Autodesk Fusion 360 part; units mm, degrees
(part 3 of 7)
sketch "スケッチ8" plane through (0, 0, 15) normal (0, 0, 1) x (-1, 0, 0)
  line L0 (-22, 92.5) -> (-17.5, 92.5)
  line L1 (-17.5, 92.5) -> (-15, 95)
  line L2 (-15, 95) -> (-10, 95)
  line L3 (-10, 95) -> (-7.5, 92.5)
  line L4 (-7.5, 92.5) -> (-3, 92.5)
  arc A0 (-3, 91.5) -> (-3, 92.5) centre (-3, 92) ccw
  line L5 (-3, 91.5) -> (-7.5, 91.5)
  line L6 (-7.5, 91.5) -> (-10, 94)
  line L7 (-10, 94) -> (-15, 94)
  line L8 (-15, 94) -> (-17.5, 91.5)
  line L9 (-17.5, 91.5) -> (-22, 91.5)
  arc A1 (-22, 92.5) -> (-22, 91.5) centre (-22, 92) ccw
  arc A2 (-9.9466, 90.4891) -> (-15.0533, 90.4891) centre (-12.5, 89.9985) ccw
  line L10 (-9.9466, 90.4891) -> (-3, 90.4891)
  arc A3 (-3, 89.508) -> (-3, 90.4891) centre (-2.9907, 89.9985) ccw
  line L11 (-3, 89.508) -> (-9.9467, 89.508)
  arc A4 (-15.0532, 89.508) -> (-9.9467, 89.508) centre (-12.5, 89.9985) ccw
  line L12 (-15.0532, 89.508) -> (-22, 89.508)
  arc A5 (-22, 90.4891) -> (-22, 89.508) centre (-22.0093, 89.9985) ccw
  line L13 (-22, 90.4891) -> (-15.0533, 90.4891)
  line L14 (-257, 90.4891) -> (-250.0533, 90.4891)
  arc A6 (-244.9466, 90.4891) -> (-250.0533, 90.4891) centre (-247.5, 89.9985) ccw
  line L15 (-244.9466, 90.4891) -> (-238, 90.4891)
  arc A7 (-238, 89.508) -> (-238, 90.4891) centre (-237.9907, 89.9985) ccw
  line L16 (-238, 89.508) -> (-244.9467, 89.508)
  arc A8 (-250.0532, 89.508) -> (-244.9467, 89.508) centre (-247.5, 89.9985) ccw
  line L17 (-250.0532, 89.508) -> (-257, 89.508)
  arc A9 (-257, 90.4891) -> (-257, 89.508) centre (-257.0093, 89.9985) ccw
  line L18 (-257, 92.5) -> (-252.5, 92.5)
  line L19 (-252.5, 92.5) -> (-250, 95)
  line L20 (-250, 95) -> (-245, 95)
  line L21 (-245, 95) -> (-242.5, 92.5)
  line L22 (-242.5, 92.5) -> (-238, 92.5)
  arc A10 (-238, 91.5) -> (-238, 92.5) centre (-238, 92) ccw
  line L23 (-238, 91.5) -> (-242.5, 91.5)
  line L24 (-242.5, 91.5) -> (-245, 94)
  line L25 (-245, 94) -> (-250, 94)
  line L26 (-250, 94) -> (-252.5, 91.5)
  line L27 (-252.5, 91.5) -> (-257, 91.5)
  arc A11 (-257, 92.5) -> (-257, 91.5) centre (-257, 92) ccw
  line L28 (-5.5, 97) -> (-254.5, 97)
  arc A12 (-254.5, 97) -> (-260.1618, 89.0141) centre (-254.5, 91) ccw
  arc A13 (-257.5, 70) -> (-260.1618, 89.0141) centre (-326.7422, 70) ccw
  spline S0 degree 3 poles (-257.5, 70) (-257.4682, 70) (-257.4042, 70.0035) (-257.3084, 70.0191) (-257.2129, 70.045) (-257.0835, 70.094) (-256.9569, 70.1632) (-256.8341, 70.249) (-256.7405, 70.3242) (-256.6475, 70.4088) (-256.555, 70.5025) (-256.4632, 70.6049) (-256.3391, 70.7561) (-256.1865, 70.9661) (-256.0102, 71.2437) (-255.8375, 71.5492) (-255.6685, 71.8799) (-255.5036, 72.2332) (-255.3429, 72.6062) (-255.1866, 72.9962) (-255.0347, 73.4004) (-254.8872, 73.8162) (-254.6952, 74.3858) (-254.4671, 75.111) (-254.2087, 75.9886) (-253.9612, 76.8646) (-253.7209, 77.7274) (-253.4836, 78.5677) (-253.2448, 79.3779) (-253, 80.1518) (-252.745, 80.8848) (-252.4757, 81.5734) (-252.189, 82.2149) (-251.8824, 82.8074) (-251.5542, 83.3498) (-251.2032, 83.8412) (-250.8288, 84.2811) (-250.4306, 84.6692) (-250.1457, 84.8961) (-250, 85) knots -1.723892 -1.723892 -1.723892 -1.723892 -1.714347 -1.704698 -1.694847 -1.684702 -1.663244 -1.65179 -1.639799 -1.627239 -1.614089 -1.600335 -1.585971 -1.555429 -1.522524 -1.487384 -1.450184 -1.411129 -1.370442 -1.328355 -1.285102 -1.240909 -1.195991 -1.104775 -1.012886 -0.921529 -0.831696 -0.744179 -0.659582 -0.578332 -0.500694 -0.426786 -0.356594 -0.289994 -0.226758 -0.166571 -0.109035 -0.053684 0 0 0 0
  spline S1 degree 5 poles (-250, 85) (-249.8618, 84.9014) (-249.5912, 84.691) (-249.2034, 84.3357) (-248.7221, 83.7824) (-248.1794, 82.9585) (-247.6925, 82.0039) (-247.2547, 80.9239) (-246.8537, 79.7274) (-246.4726, 78.4298) (-246.0928, 77.0547) (-245.6957, 75.6366) (-245.2655, 74.223) (-244.7912, 72.8764) (-244.2698, 71.6789) (-243.7063, 70.7262) (-243.1114, 70.1082) (-242.5, 69.8927) (-241.8886, 70.1082) (-241.2937, 70.7262) (-240.7302, 71.6789) (-240.2088, 72.8764) (-239.7345, 74.223) (-239.3043, 75.6366) (-238.9072, 77.0547) (-238.5274, 78.4298) (-238.1463, 79.7274) (-237.7453, 80.9239) (-237.3075, 82.0039) (-236.8206, 82.9585) (-236.2779, 83.7824) (-235.7966, 84.3357) (-235.4088, 84.691) (-235.1382, 84.9014) (-235, 85) knots -1 -1 -1 -1 -1 -1 -0.966667 -0.933333 -0.9 -0.866667 -0.833333 -0.8 -0.766667 -0.733333 -0.7 -0.666667 -0.633333 -0.6 -0.566667 -0.533333 -0.5 -0.466667 -0.433333 -0.4 -0.366667 -0.333333 -0.3 -0.266667 -0.233333 -0.2 -0.166667 -0.133333 -0.1 -0.066667 -0.033333 0 0 0 0 0 0
  spline S2 degree 5 poles (-235, 85) (-234.8618, 84.9014) (-234.5912, 84.691) (-234.2034, 84.3357) (-233.7221, 83.7824) (-233.1794, 82.9585) (-232.6925, 82.0039) (-232.2547, 80.9239) (-231.8537, 79.7274) (-231.4726, 78.4298) (-231.0928, 77.0547) (-230.6957, 75.6366) (-230.2655, 74.223) (-229.7912, 72.8764) (-229.2698, 71.6789) (-228.7063, 70.7262) (-228.1114, 70.1082) (-227.5, 69.8927) (-226.8886, 70.1082) (-226.2937, 70.7262) (-225.7302, 71.6789) (-225.2088, 72.8764) (-224.7345, 74.223) (-224.3043, 75.6366) (-223.9072, 77.0547) (-223.5274, 78.4298) (-223.1463, 79.7274) (-222.7453, 80.9239) (-222.3075, 82.0039) (-221.8206, 82.9585) (-221.2779, 83.7824) (-220.7966, 84.3357) (-220.4088, 84.691) (-220.1382, 84.9014) (-220, 85) knots -1 -1 -1 -1 -1 -1 -0.966667 -0.933333 -0.9 -0.866667 -0.833333 -0.8 -0.766667 -0.733333 -0.7 -0.666667 -0.633333 -0.6 -0.566667 -0.533333 -0.5 -0.466667 -0.433333 -0.4 -0.366667 -0.333333 -0.3 -0.266667 -0.233333 -0.2 -0.166667 -0.133333 -0.1 -0.066667 -0.033333 0 0 0 0 0 0
  spline S3 degree 5 poles (-220, 85) (-219.8618, 84.9014) (-219.5912, 84.691) (-219.2034, 84.3357) (-218.7221, 83.7824) (-218.1794, 82.9585) (-217.6925, 82.0039) (-217.2547, 80.9239) (-216.8537, 79.7274) (-216.4726, 78.4298) (-216.0928, 77.0547) (-215.6957, 75.6366) (-215.2655, 74.223) (-214.7912, 72.8764) (-214.2698, 71.6789) (-213.7063, 70.7262) (-213.1114, 70.1082) (-212.5, 69.8927) (-211.8886, 70.1082) (-211.2937, 70.7262) (-210.7302, 71.6789) (-210.2088, 72.8764) (-209.7345, 74.223) (-209.3043, 75.6366) (-208.9072, 77.0547) (-208.5274, 78.4298) (-208.1463, 79.7274) (-207.7453, 80.9239) (-207.3075, 82.0039) (-206.8206, 82.9585) (-206.2779, 83.7824) (-205.7966, 84.3357) (-205.4088, 84.691) (-205.1382, 84.9014) (-205, 85) knots -1 -1 -1 -1 -1 -1 -0.966667 -0.933333 -0.9 -0.866667 -0.833333 -0.8 -0.766667 -0.733333 -0.7 -0.666667 -0.633333 -0.6 -0.566667 -0.533333 -0.5 -0.466667 -0.433333 -0.4 -0.366667 -0.333333 -0.3 -0.266667 -0.233333 -0.2 -0.166667 -0.133333 -0.1 -0.066667 -0.033333 0 0 0 0 0 0
  spline S4 degree 5 poles (-205, 85) (-204.8618, 84.9014) (-204.5912, 84.691) (-204.2034, 84.3357) (-203.7221, 83.7824) (-203.1794, 82.9585) (-202.6925, 82.0039) (-202.2547, 80.9239) (-201.8537, 79.7274) (-201.4726, 78.4298) (-201.0928, 77.0547) (-200.6957, 75.6366) (-200.2655, 74.223) (-199.7912, 72.8764) (-199.2698, 71.6789) (-198.7063, 70.7262) (-198.1114, 70.1082) (-197.5, 69.8927) (-196.8886, 70.1082) (-196.2937, 70.7262) (-195.7302, 71.6789) (-195.2088, 72.8764) (-194.7345, 74.223) (-194.3043, 75.6366) (-193.9072, 77.0547) (-193.5274, 78.4298) (-193.1463, 79.7274) (-192.7453, 80.9239) (-192.3075, 82.0039) (-191.8206, 82.9585) (-191.2779, 83.7824) (-190.7966, 84.3357) (-190.4088, 84.691) (-190.1382, 84.9014) (-190, 85) knots -1 -1 -1 -1 -1 -1 -0.966667 -0.933333 -0.9 -0.866667 -0.833333 -0.8 -0.766667 -0.733333 -0.7 -0.666667 -0.633333 -0.6 -0.566667 -0.533333 -0.5 -0.466667 -0.433333 -0.4 -0.366667 -0.333333 -0.3 -0.266667 -0.233333 -0.2 -0.166667 -0.133333 -0.1 -0.066667 -0.033333 0 0 0 0 0 0
  spline S5 degree 5 poles (-190, 85) (-189.8618, 84.9014) (-189.5912, 84.691) (-189.2034, 84.3357) (-188.7221, 83.7824) (-188.1794, 82.9585) (-187.6925, 82.0039) (-187.2547, 80.9239) (-186.8537, 79.7274) (-186.4726, 78.4298) (-186.0928, 77.0547) (-185.6957, 75.6366) (-185.2655, 74.223) (-184.7912, 72.8764) (-184.2698, 71.6789) (-183.7063, 70.7262) (-183.1114, 70.1082) (-182.5, 69.8927) (-181.8886, 70.1082) (-181.2937, 70.7262) (-180.7302, 71.6789) (-180.2088, 72.8764) (-179.7345, 74.223) (-179.3043, 75.6366) (-178.9072, 77.0547) (-178.5274, 78.4298) (-178.1463, 79.7274) (-177.7453, 80.9239) (-177.3075, 82.0039) (-176.8206, 82.9585) (-176.2779, 83.7824) (-175.7966, 84.3357) (-175.4088, 84.691) (-175.1382, 84.9014) (-175, 85) knots -1 -1 -1 -1 -1 -1 -0.966667 -0.933333 -0.9 -0.866667 -0.833333 -0.8 -0.766667 -0.733333 -0.7 -0.666667 -0.633333 -0.6 -0.566667 -0.533333 -0.5 -0.466667 -0.433333 -0.4 -0.366667 -0.333333 -0.3 -0.266667 -0.233333 -0.2 -0.166667 -0.133333 -0.1 -0.066667 -0.033333 0 0 0 0 0 0
  spline S6 degree 5 poles (-175, 85) (-174.8618, 84.9014) (-174.5912, 84.691) (-174.2034, 84.3357) (-173.7221, 83.7824) (-173.1794, 82.9585) (-172.6925, 82.0039) (-172.2547, 80.9239) (-171.8537, 79.7274) (-171.4726, 78.4298) (-171.0928, 77.0547) (-170.6957, 75.6366) (-170.2655, 74.223) (-169.7912, 72.8764) (-169.2698, 71.6789) (-168.7063, 70.7262) (-168.1114, 70.1082) (-167.5, 69.8927) (-166.8886, 70.1082) (-166.2937, 70.7262) (-165.7302, 71.6789) (-165.2088, 72.8764) (-164.7345, 74.223) (-164.3043, 75.6366) (-163.9072, 77.0547) (-163.5274, 78.4298) (-163.1463, 79.7274) (-162.7453, 80.9239) (-162.3075, 82.0039) (-161.8206, 82.9585) (-161.2779, 83.7824) (-160.7966, 84.3357) (-160.4088, 84.691) (-160.1382, 84.9014) (-160, 85) knots -1 -1 -1 -1 -1 -1 -0.966667 -0.933333 -0.9 -0.866667 -0.833333 -0.8 -0.766667 -0.733333 -0.7 -0.666667 -0.633333 -0.6 -0.566667 -0.533333 -0.5 -0.466667 -0.433333 -0.4 -0.366667 -0.333333 -0.3 -0.266667 -0.233333 -0.2 -0.166667 -0.133333 -0.1 -0.066667 -0.033333 0 0 0 0 0 0
  spline S7 degree 5 poles (-160, 85) (-159.8618, 84.9014) (-159.5912, 84.691) (-159.2034, 84.3357) (-158.7221, 83.7824) (-158.1794, 82.9585) (-157.6925, 82.0039) (-157.2547, 80.9239) (-156.8537, 79.7274) (-156.4726, 78.4298) (-156.0928, 77.0547) (-155.6957, 75.6366) (-155.2655, 74.223) (-154.7912, 72.8764) (-154.2698, 71.6789) (-153.7063, 70.7262) (-153.1114, 70.1082) (-152.5, 69.8927) (-151.8886, 70.1082) (-151.2937, 70.7262) (-150.7302, 71.6789) (-150.2088, 72.8764) (-149.7345, 74.223) (-149.3043, 75.6366) (-148.9072, 77.0547) (-148.5274, 78.4298) (-148.1463, 79.7274) (-147.7453, 80.9239) (-147.3075, 82.0039) (-146.8206, 82.9585) (-146.2779, 83.7824) (-145.7966, 84.3357) (-145.4088, 84.691) (-145.1382, 84.9014) (-145, 85) knots -1 -1 -1 -1 -1 -1 -0.966667 -0.933333 -0.9 -0.866667 -0.833333 -0.8 -0.766667 -0.733333 -0.7 -0.666667 -0.633333 -0.6 -0.566667 -0.533333 -0.5 -0.466667 -0.433333 -0.4 -0.366667 -0.333333 -0.3 -0.266667 -0.233333 -0.2 -0.166667 -0.133333 -0.1 -0.066667 -0.033333 0 0 0 0 0 0
  spline S8 degree 5 poles (-145, 85) (-144.8618, 84.9014) (-144.5912, 84.691) (-144.2034, 84.3357) (-143.7221, 83.7824) (-143.1794, 82.9585) (-142.6925, 82.0039) (-142.2547, 80.9239) (-141.8537, 79.7274) (-141.4726, 78.4298) (-141.0928, 77.0547) (-140.6957, 75.6366) (-140.2655, 74.223) (-139.7912, 72.8764) (-139.2698, 71.6789) (-138.7063, 70.7262) (-138.1114, 70.1082) (-137.5, 69.8927) (-136.8886, 70.1082) (-136.2937, 70.7262) (-135.7302, 71.6789) (-135.2088, 72.8764) (-134.7345, 74.223) (-134.3043, 75.6366) (-133.9072, 77.0547) (-133.5274, 78.4298) (-133.1463, 79.7274) (-132.7453, 80.9239) (-132.3075, 82.0039) (-131.8206, 82.9585) (-131.2779, 83.7824) (-130.7966, 84.3357) (-130.4088, 84.691) (-130.1382, 84.9014) (-130, 85) knots -1 -1 -1 -1 -1 -1 -0.966667 -0.933333 -0.9 -0.866667 -0.833333 -0.8 -0.766667 -0.733333 -0.7 -0.666667 -0.633333 -0.6 -0.566667 -0.533333 -0.5 -0.466667 -0.433333 -0.4 -0.366667 -0.333333 -0.3 -0.266667 -0.233333 -0.2 -0.166667 -0.133333 -0.1 -0.066667 -0.033333 0 0 0 0 0 0
  spline S9 degree 5 poles (-130, 85) (-129.8618, 84.9014) (-129.5912, 84.691) (-129.2034, 84.3357) (-128.7221, 83.7824) (-128.1794, 82.9585) (-127.6925, 82.0039) (-127.2547, 80.9239) (-126.8537, 79.7274) (-126.4726, 78.4298) (-126.0928, 77.0547) (-125.6957, 75.6366) (-125.2655, 74.223) (-124.7912, 72.8764) (-124.2698, 71.6789) (-123.7063, 70.7262) (-123.1114, 70.1082) (-122.5, 69.8927) (-121.8886, 70.1082) (-121.2937, 70.7262) (-120.7302, 71.6789) (-120.2088, 72.8764) (-119.7345, 74.223) (-119.3043, 75.6366) (-118.9072, 77.0547) (-118.5274, 78.4298) (-118.1463, 79.7274) (-117.7453, 80.9239) (-117.3075, 82.0039) (-116.8206, 82.9585) (-116.2779, 83.7824) (-115.7966, 84.3357) (-115.4088, 84.691) (-115.1382, 84.9014) (-115, 85) knots -1 -1 -1 -1 -1 -1 -0.966667 -0.933333 -0.9 -0.866667 -0.833333 -0.8 -0.766667 -0.733333 -0.7 -0.666667 -0.633333 -0.6 -0.566667 -0.533333 -0.5 -0.466667 -0.433333 -0.4 -0.366667 -0.333333 -0.3 -0.266667 -0.233333 -0.2 -0.166667 -0.133333 -0.1 -0.066667 -0.033333 0 0 0 0 0 0
  spline S10 degree 5 poles (-115, 85) (-114.8618, 84.9014) (-114.5912, 84.691) (-114.2034, 84.3357) (-113.7221, 83.7824) (-113.1794, 82.9585) (-112.6925, 82.0039) (-112.2547, 80.9239) (-111.8537, 79.7274) (-111.4726, 78.4298) (-111.0928, 77.0547) (-110.6957, 75.6366) (-110.2655, 74.223) (-109.7912, 72.8764) (-109.2698, 71.6789) (-108.7063, 70.7262) (-108.1114, 70.1082) (-107.5, 69.8927) (-106.8886, 70.1082) (-106.2937, 70.7262) (-105.7302, 71.6789) (-105.2088, 72.8764) (-104.7345, 74.223) (-104.3043, 75.6366) (-103.9072, 77.0547) (-103.5274, 78.4298) (-103.1463, 79.7274) (-102.7453, 80.9239) (-102.3075, 82.0039) (-101.8206, 82.9585) (-101.2779, 83.7824) (-100.7966, 84.3357) (-100.4088, 84.691) (-100.1382, 84.9014) (-100, 85) knots -1 -1 -1 -1 -1 -1 -0.966667 -0.933333 -0.9 -0.866667 -0.833333 -0.8 -0.766667 -0.733333 -0.7 -0.666667 -0.633333 -0.6 -0.566667 -0.533333 -0.5 -0.466667 -0.433333 -0.4 -0.366667 -0.333333 -0.3 -0.266667 -0.233333 -0.2 -0.166667 -0.133333 -0.1 -0.066667 -0.033333 0 0 0 0 0 0
  spline S11 degree 5 poles (-100, 85) (-99.8618, 84.9014) (-99.5912, 84.691) (-99.2034, 84.3357) (-98.7221, 83.7824) (-98.1794, 82.9585) (-97.6925, 82.0039) (-97.2547, 80.9239) (-96.8537, 79.7274) (-96.4726, 78.4298) (-96.0928, 77.0547) (-95.6957, 75.6366) (-95.2655, 74.223) (-94.7912, 72.8764) (-94.2698, 71.6789) (-93.7063, 70.7262) (-93.1114, 70.1082) (-92.5, 69.8927) (-91.8886, 70.1082) (-91.2937, 70.7262) (-90.7302, 71.6789) (-90.2088, 72.8764) (-89.7345, 74.223) (-89.3043, 75.6366) (-88.9072, 77.0547) (-88.5274, 78.4298) (-88.1463, 79.7274) (-87.7453, 80.9239) (-87.3075, 82.0039) (-86.8206, 82.9585) (-86.2779, 83.7824) (-85.7966, 84.3357) (-85.4088, 84.691) (-85.1382, 84.9014) (-85, 85) knots -1 -1 -1 -1 -1 -1 -0.966667 -0.933333 -0.9 -0.866667 -0.833333 -0.8 -0.766667 -0.733333 -0.7 -0.666667 -0.633333 -0.6 -0.566667 -0.533333 -0.5 -0.466667 -0.433333 -0.4 -0.366667 -0.333333 -0.3 -0.266667 -0.233333 -0.2 -0.166667 -0.133333 -0.1 -0.066667 -0.033333 0 0 0 0 0 0
  spline S12 degree 5 poles (-85, 85) (-84.8618, 84.9014) (-84.5912, 84.691) (-84.2034, 84.3357) (-83.7221, 83.7824) (-83.1794, 82.9585) (-82.6925, 82.0039) (-82.2547, 80.9239) (-81.8537, 79.7274) (-81.4726, 78.4298) (-81.0928, 77.0547) (-80.6957, 75.6366) (-80.2655, 74.223) (-79.7912, 72.8764) (-79.2698, 71.6789) (-78.7063, 70.7262) (-78.1114, 70.1082) (-77.5, 69.8927) (-76.8886, 70.1082) (-76.2937, 70.7262) (-75.7302, 71.6789) (-75.2088, 72.8764) (-74.7345, 74.223) (-74.3043, 75.6366) (-73.9072, 77.0547) (-73.5274, 78.4298) (-73.1463, 79.7274) (-72.7453, 80.9239) (-72.3075, 82.0039) (-71.8206, 82.9585) (-71.2779, 83.7824) (-70.7966, 84.3357) (-70.4088, 84.691) (-70.1382, 84.9014) (-70, 85) knots -1 -1 -1 -1 -1 -1 -0.966667 -0.933333 -0.9 -0.866667 -0.833333 -0.8 -0.766667 -0.733333 -0.7 -0.666667 -0.633333 -0.6 -0.566667 -0.533333 -0.5 -0.466667 -0.433333 -0.4 -0.366667 -0.333333 -0.3 -0.266667 -0.233333 -0.2 -0.166667 -0.133333 -0.1 -0.066667 -0.033333 0 0 0 0 0 0
  spline S13 degree 5 poles (-70, 85) (-69.8618, 84.9014) (-69.5912, 84.691) (-69.2034, 84.3357) (-68.7221, 83.7824) (-68.1794, 82.9585) (-67.6925, 82.0039) (-67.2547, 80.9239) (-66.8537, 79.7274) (-66.4726, 78.4298) (-66.0928, 77.0547) (-65.6957, 75.6366) (-65.2655, 74.223) (-64.7912, 72.8764) (-64.2698, 71.6789) (-63.7063, 70.7262) (-63.1114, 70.1082) (-62.5, 69.8927) (-61.8886, 70.1082) (-61.2937, 70.7262) (-60.7302, 71.6789) (-60.2088, 72.8764) (-59.7345, 74.223) (-59.3043, 75.6366) (-58.9072, 77.0547) (-58.5274, 78.4298) (-58.1463, 79.7274) (-57.7453, 80.9239) (-57.3075, 82.0039) (-56.8206, 82.9585) (-56.2779, 83.7824) (-55.7966, 84.3357) (-55.4088, 84.691) (-55.1382, 84.9014) (-55, 85) knots -1 -1 -1 -1 -1 -1 -0.966667 -0.933333 -0.9 -0.866667 -0.833333 -0.8 -0.766667 -0.733333 -0.7 -0.666667 -0.633333 -0.6 -0.566667 -0.533333 -0.5 -0.466667 -0.433333 -0.4 -0.366667 -0.333333 -0.3 -0.266667 -0.233333 -0.2 -0.166667 -0.133333 -0.1 -0.066667 -0.033333 0 0 0 0 0 0
  spline S14 degree 5 poles (-55, 85) (-54.8618, 84.9014) (-54.5912, 84.691) (-54.2034, 84.3357) (-53.7221, 83.7824) (-53.1794, 82.9585) (-52.6925, 82.0039) (-52.2547, 80.9239) (-51.8537, 79.7274) (-51.4726, 78.4298) (-51.0928, 77.0547) (-50.6957, 75.6366) (-50.2655, 74.223) (-49.7912, 72.8764) (-49.2698, 71.6789) (-48.7063, 70.7262) (-48.1114, 70.1082) (-47.5, 69.8927) (-46.8886, 70.1082) (-46.2937, 70.7262) (-45.7302, 71.6789) (-45.2088, 72.8764) (-44.7345, 74.223) (-44.3043, 75.6366) (-43.9072, 77.0547) (-43.5274, 78.4298) (-43.1463, 79.7274) (-42.7453, 80.9239) (-42.3075, 82.0039) (-41.8206, 82.9585) (-41.2779, 83.7824) (-40.7966, 84.3357) (-40.4088, 84.691) (-40.1382, 84.9014) (-40, 85) knots -1 -1 -1 -1 -1 -1 -0.966667 -0.933333 -0.9 -0.866667 -0.833333 -0.8 -0.766667 -0.733333 -0.7 -0.666667 -0.633333 -0.6 -0.566667 -0.533333 -0.5 -0.466667 -0.433333 -0.4 -0.366667 -0.333333 -0.3 -0.266667 -0.233333 -0.2 -0.166667 -0.133333 -0.1 -0.066667 -0.033333 0 0 0 0 0 0
  spline S15 degree 5 poles (-40, 85) (-39.8618, 84.9014) (-39.5912, 84.691) (-39.2034, 84.3357) (-38.7221, 83.7824) (-38.1794, 82.9585) (-37.6925, 82.0039) (-37.2547, 80.9239) (-36.8537, 79.7274) (-36.4726, 78.4298) (-36.0928, 77.0547) (-35.6957, 75.6366) (-35.2655, 74.223) (-34.7912, 72.8764) (-34.2698, 71.6789) (-33.7063, 70.7262) (-33.1114, 70.1082) (-32.5, 69.8927) (-31.8886, 70.1082) (-31.2937, 70.7262) (-30.7302, 71.6789) (-30.2088, 72.8764) (-29.7345, 74.223) (-29.3043, 75.6366) (-28.9072, 77.0547) (-28.5274, 78.4298) (-28.1463, 79.7274) (-27.7453, 80.9239) (-27.3075, 82.0039) (-26.8206, 82.9585) (-26.2779, 83.7824) (-25.7966, 84.3357) (-25.4088, 84.691) (-25.1382, 84.9014) (-25, 85) knots -1 -1 -1 -1 -1 -1 -0.966667 -0.933333 -0.9 -0.866667 -0.833333 -0.8 -0.766667 -0.733333 -0.7 -0.666667 -0.633333 -0.6 -0.566667 -0.533333 -0.5 -0.466667 -0.433333 -0.4 -0.366667 -0.333333 -0.3 -0.266667 -0.233333 -0.2 -0.166667 -0.133333 -0.1 -0.066667 -0.033333 0 0 0 0 0 0
  spline S16 degree 5 poles (-25, 85) (-24.8618, 84.9014) (-24.5912, 84.691) (-24.2034, 84.3357) (-23.7221, 83.7824) (-23.1794, 82.9585) (-22.6925, 82.0039) (-22.2547, 80.9239) (-21.8537, 79.7274) (-21.4726, 78.4298) (-21.0928, 77.0547) (-20.6957, 75.6366) (-20.2655, 74.223) (-19.7912, 72.8764) (-19.2698, 71.6789) (-18.7063, 70.7262) (-18.1114, 70.1082) (-17.5, 69.8927) (-16.8886, 70.1082) (-16.2937, 70.7262) (-15.7302, 71.6789) (-15.2088, 72.8764) (-14.7345, 74.223) (-14.3043, 75.6366) (-13.9072, 77.0547) (-13.5274, 78.4298) (-13.1463, 79.7274) (-12.7453, 80.9239) (-12.3075, 82.0039) (-11.8206, 82.9585) (-11.2779, 83.7824) (-10.7966, 84.3357) (-10.4088, 84.691) (-10.1382, 84.9014) (-10, 85) knots -1 -1 -1 -1 -1 -1 -0.966667 -0.933333 -0.9 -0.866667 -0.833333 -0.8 -0.766667 -0.733333 -0.7 -0.666667 -0.633333 -0.6 -0.566667 -0.533333 -0.5 -0.466667 -0.433333 -0.4 -0.366667 -0.333333 -0.3 -0.266667 -0.233333 -0.2 -0.166667 -0.133333 -0.1 -0.066667 -0.033333 0 0 0 0 0 0
  spline S17 degree 5 poles (-10, 85) (-9.8618, 84.9014) (-9.5912, 84.691) (-9.2034, 84.3357) (-8.7221, 83.7824) (-8.1794, 82.9585) (-7.6925, 82.0039) (-7.2547, 80.9239) (-6.8537, 79.7274) (-6.4726, 78.4298) (-6.0928, 77.0547) (-5.6957, 75.6366) (-5.2655, 74.223) (-4.7912, 72.8764) (-4.2698, 71.6789) (-3.7063, 70.7262) (-3.2304, 70.2318) (-2.866, 70.0421) (-2.622, 70) (-2.5, 70) knots -1 -1 -1 -1 -1 -1 -0.966667 -0.933333 -0.9 -0.866667 -0.833333 -0.8 -0.766667 -0.733333 -0.7 -0.666667 -0.633333 -0.6 -0.566667 -0.533333 -0.5 -0.5 -0.5 -0.5 -0.5 -0.5
  arc A14 (-0.0354, 88.5224) -> (-2.5, 70) centre (93.3503, 66.6714) ccw
  arc A15 (-0.0354, 88.5224) -> (-5.5, 97) centre (-5.5, 91) ccw
  spline S18 degree 3 poles (-40, 87.4565) (-39.6129, 87.1804) (-39.2258, 86.9044) (-38.8387, 86.6283) (-37.4048, 85.6057) (-36.3881, 84.0523) (-35.6468, 82.2521) (-34.9554, 80.5733) (-34.4675, 78.6373) (-33.9195, 76.7225) (-33.5808, 75.5389) (-33.2149, 74.3638) (-32.8326, 73.4325) (-32.7208, 73.1603) (-32.6088, 72.9111) (-32.5, 72.6931) knots -1.056001 -1.056001 -1.056001 -1.056001 -1 -1 -1 -0.851292 -0.851292 -0.851292 -0.71262 -0.71262 -0.71262 -0.626906 -0.626906 -0.626906 -0.601856 -0.601856 -0.601856 -0.601856
  spline S19 degree 3 poles (-32.5, 72.6931) (-32.0881, 73.5183) (-31.6514, 74.7828) (-31.2668, 76.0817) (-30.7129, 77.9522) (-30.237, 79.9069) (-29.6002, 81.6203) (-28.9085, 83.4814) (-27.986, 85.1149) (-26.6355, 86.2591) (-26.4823, 86.3889) (-26.3242, 86.5122) (-26.1613, 86.6283) (-25.7742, 86.9044) (-25.3871, 87.1804) (-25, 87.4565) knots -0.398144 -0.398144 -0.398144 -0.398144 -0.30293 -0.30293 -0.30293 -0.165823 -0.165823 -0.165823 -0.016893 -0.016893 -0.016893 0 0 0 0.056001 0.056001 0.056001 0.056001
  spline S20 degree 3 poles (-25, 87.4565) (-24.6129, 87.1804) (-24.2258, 86.9044) (-23.8387, 86.6283) (-22.4048, 85.6057) (-21.3881, 84.0523) (-20.6468, 82.2521) (-19.9554, 80.5733) (-19.4675, 78.6373) (-18.9195, 76.7225) (-18.5808, 75.5389) (-18.2149, 74.3638) (-17.8326, 73.4325) (-17.7208, 73.1603) (-17.6088, 72.9111) (-17.5, 72.6931) knots -1.056001 -1.056001 -1.056001 -1.056001 -1 -1 -1 -0.851292 -0.851292 -0.851292 -0.71262 -0.71262 -0.71262 -0.626906 -0.626906 -0.626906 -0.601856 -0.601856 -0.601856 -0.601856
  arc A16 (-2.3166, 87.5) -> (-4.0079, 77.0332) centre (93.3503, 66.6714) ccw
  arc A17 (-255.8863, 77.4088) -> (-257.6718, 87.4565) centre (-326.7422, 70) ccw
  spline S21 degree 3 poles (-242.5, 72.6931) (-242.0881, 73.5183) (-241.6514, 74.7828) (-241.2668, 76.0817) (-240.7129, 77.9522) (-240.237, 79.9069) (-239.6002, 81.6203) (-238.9085, 83.4814) (-237.986, 85.1149) (-236.6355, 86.2591) (-236.4823, 86.3889) (-236.3242, 86.5122) (-236.1613, 86.6283) (-235.7742, 86.9044) (-235.3871, 87.1804) (-235, 87.4565) knots -0.398144 -0.398144 -0.398144 -0.398144 -0.30293 -0.30293 -0.30293 -0.165823 -0.165823 -0.165823 -0.016893 -0.016893 -0.016893 0 0 0 0.056001 0.056001 0.056001 0.056001
  spline S22 degree 3 poles (-235, 87.4565) (-234.6129, 87.1804) (-234.2258, 86.9044) (-233.8387, 86.6283) (-232.4048, 85.6057) (-231.3881, 84.0523) (-230.6468, 82.2521) (-229.9554, 80.5733) (-229.4675, 78.6373) (-228.9195, 76.7225) (-228.5808, 75.5389) (-228.2149, 74.3638) (-227.8326, 73.4325) (-227.7208, 73.1603) (-227.6088, 72.9111) (-227.5, 72.6931) knots -1.056001 -1.056001 -1.056001 -1.056001 -1 -1 -1 -0.851292 -0.851292 -0.851292 -0.71262 -0.71262 -0.71262 -0.626906 -0.626906 -0.626906 -0.601856 -0.601856 -0.601856 -0.601856
  spline S23 degree 3 poles (-227.5, 72.6931) (-227.0881, 73.5183) (-226.6514, 74.7828) (-226.2668, 76.0817) (-225.7129, 77.9522) (-225.237, 79.9069) (-224.6002, 81.6203) (-223.9085, 83.4814) (-222.986, 85.1149) (-221.6355, 86.2591) (-221.4823, 86.3889) (-221.3242, 86.5122) (-221.1613, 86.6283) (-220.7742, 86.9044) (-220.3871, 87.1804) (-220, 87.4565) knots -0.398144 -0.398144 -0.398144 -0.398144 -0.30293 -0.30293 -0.30293 -0.165823 -0.165823 -0.165823 -0.016893 -0.016893 -0.016893 0 0 0 0.056001 0.056001 0.056001 0.056001
  spline S24 degree 3 poles (-220, 87.4565) (-219.6129, 87.1804) (-219.2258, 86.9044) (-218.8387, 86.6283) (-217.4048, 85.6057) (-216.3881, 84.0523) (-215.6468, 82.2521) (-214.9554, 80.5733) (-214.4675, 78.6373) (-213.9195, 76.7225) (-213.5808, 75.5389) (-213.2149, 74.3638) (-212.8326, 73.4325) (-212.7208, 73.1603) (-212.6088, 72.9111) (-212.5, 72.6931) knots -1.056001 -1.056001 -1.056001 -1.056001 -1 -1 -1 -0.851292 -0.851292 -0.851292 -0.71262 -0.71262 -0.71262 -0.626906 -0.626906 -0.626906 -0.601856 -0.601856 -0.601856 -0.601856
  spline S25 degree 3 poles (-212.5, 72.6931) (-212.0881, 73.5183) (-211.6514, 74.7828) (-211.2668, 76.0817) (-210.7129, 77.9522) (-210.237, 79.9069) (-209.6002, 81.6203) (-208.9085, 83.4814) (-207.986, 85.1149) (-206.6355, 86.2591) (-206.4823, 86.3889) (-206.3242, 86.5122) (-206.1613, 86.6283) (-205.7742, 86.9044) (-205.3871, 87.1804) (-205, 87.4565) knots -0.398144 -0.398144 -0.398144 -0.398144 -0.30293 -0.30293 -0.30293 -0.165823 -0.165823 -0.165823 -0.016893 -0.016893 -0.016893 0 0 0 0.056001 0.056001 0.056001 0.056001
  spline S26 degree 3 poles (-205, 87.4565) (-204.6129, 87.1804) (-204.2258, 86.9044) (-203.8387, 86.6283) (-202.4048, 85.6057) (-201.3881, 84.0523) (-200.6468, 82.2521) (-199.9554, 80.5733) (-199.4675, 78.6373) (-198.9195, 76.7225) (-198.5808, 75.5389) (-198.2149, 74.3638) (-197.8326, 73.4325) (-197.7208, 73.1603) (-197.6088, 72.9111) (-197.5, 72.6931) knots -1.056001 -1.056001 -1.056001 -1.056001 -1 -1 -1 -0.851292 -0.851292 -0.851292 -0.71262 -0.71262 -0.71262 -0.626906 -0.626906 -0.626906 -0.601856 -0.601856 -0.601856 -0.601856
  spline S27 degree 3 poles (-197.5, 72.6931) (-197.0881, 73.5183) (-196.6514, 74.7828) (-196.2668, 76.0817) (-195.7129, 77.9522) (-195.237, 79.9069) (-194.6002, 81.6203) (-193.9085, 83.4814) (-192.986, 85.1149) (-191.6355, 86.2591) (-191.4823, 86.3889) (-191.3242, 86.5122) (-191.1613, 86.6283) (-190.7742, 86.9044) (-190.3871, 87.1804) (-190, 87.4565) knots -0.398144 -0.398144 -0.398144 -0.398144 -0.30293 -0.30293 -0.30293 -0.165823 -0.165823 -0.165823 -0.016893 -0.016893 -0.016893 0 0 0 0.056001 0.056001 0.056001 0.056001
  spline S28 degree 3 poles (-190, 87.4565) (-189.6129, 87.1804) (-189.2258, 86.9044) (-188.8387, 86.6283) (-187.4048, 85.6057) (-186.3881, 84.0523) (-185.6468, 82.2521) (-184.9554, 80.5733) (-184.4675, 78.6373) (-183.9195, 76.7225) (-183.5808, 75.5389) (-183.2149, 74.3638) (-182.8326, 73.4325) (-182.7208, 73.1603) (-182.6088, 72.9111) (-182.5, 72.6931) knots -1.056001 -1.056001 -1.056001 -1.056001 -1 -1 -1 -0.851292 -0.851292 -0.851292 -0.71262 -0.71262 -0.71262 -0.626906 -0.626906 -0.626906 -0.601856 -0.601856 -0.601856 -0.601856
  spline S29 degree 3 poles (-182.5, 72.6931) (-182.0881, 73.5183) (-181.6514, 74.7828) (-181.2668, 76.0817) (-180.7129, 77.9522) (-180.237, 79.9069) (-179.6002, 81.6203) (-178.9085, 83.4814) (-177.986, 85.1149) (-176.6355, 86.2591) (-176.4823, 86.3889) (-176.3242, 86.5122) (-176.1613, 86.6283) (-175.7742, 86.9044) (-175.3871, 87.1804) (-175, 87.4565) knots -0.398144 -0.398144 -0.398144 -0.398144 -0.30293 -0.30293 -0.30293 -0.165823 -0.165823 -0.165823 -0.016893 -0.016893 -0.016893 0 0 0 0.056001 0.056001 0.056001 0.056001
  spline S30 degree 3 poles (-175, 87.4565) (-174.6129, 87.1804) (-174.2258, 86.9044) (-173.8387, 86.6283) (-172.4048, 85.6057) (-171.3881, 84.0523) (-170.6468, 82.2521) (-169.9554, 80.5733) (-169.4675, 78.6373) (-168.9195, 76.7225) (-168.5808, 75.5389) (-168.2149, 74.3638) (-167.8326, 73.4325) (-167.7208, 73.1603) (-167.6088, 72.9111) (-167.5, 72.6931) knots -1.056001 -1.056001 -1.056001 -1.056001 -1 -1 -1 -0.851292 -0.851292 -0.851292 -0.71262 -0.71262 -0.71262 -0.626906 -0.626906 -0.626906 -0.601856 -0.601856 -0.601856 -0.601856
  spline S31 degree 3 poles (-167.5, 72.6931) (-167.0881, 73.5183) (-166.6514, 74.7828) (-166.2668, 76.0817) (-165.7129, 77.9522) (-165.237, 79.9069) (-164.6002, 81.6203) (-163.9085, 83.4814) (-162.986, 85.1149) (-161.6355, 86.2591) (-161.4823, 86.3889) (-161.3242, 86.5122) (-161.1613, 86.6283) (-160.7742, 86.9044) (-160.3871, 87.1804) (-160, 87.4565) knots -0.398144 -0.398144 -0.398144 -0.398144 -0.30293 -0.30293 -0.30293 -0.165823 -0.165823 -0.165823 -0.016893 -0.016893 -0.016893 0 0 0 0.056001 0.056001 0.056001 0.056001
  spline S32 degree 3 poles (-160, 87.4565) (-159.6129, 87.1804) (-159.2258, 86.9044) (-158.8387, 86.6283) (-157.4048, 85.6057) (-156.3881, 84.0523) (-155.6468, 82.2521) (-154.9554, 80.5733) (-154.4675, 78.6373) (-153.9195, 76.7225) (-153.5808, 75.5389) (-153.2149, 74.3638) (-152.8326, 73.4325) (-152.7208, 73.1603) (-152.6088, 72.9111) (-152.5, 72.6931) knots -1.056001 -1.056001 -1.056001 -1.056001 -1 -1 -1 -0.851292 -0.851292 -0.851292 -0.71262 -0.71262 -0.71262 -0.626906 -0.626906 -0.626906 -0.601856 -0.601856 -0.601856 -0.601856
  spline S33 degree 3 poles (-152.5, 72.6931) (-152.0881, 73.5183) (-151.6514, 74.7828) (-151.2668, 76.0817) (-150.7129, 77.9522) (-150.237, 79.9069) (-149.6002, 81.6203) (-148.9085, 83.4814) (-147.986, 85.1149) (-146.6355, 86.2591) (-146.4823, 86.3889) (-146.3242, 86.5122) (-146.1613, 86.6283) (-145.7742, 86.9044) (-145.3871, 87.1804) (-145, 87.4565) knots -0.398144 -0.398144 -0.398144 -0.398144 -0.30293 -0.30293 -0.30293 -0.165823 -0.165823 -0.165823 -0.016893 -0.016893 -0.016893 0 0 0 0.056001 0.056001 0.056001 0.056001
  spline S34 degree 3 poles (-145, 87.4565) (-144.6129, 87.1804) (-144.2258, 86.9044) (-143.8387, 86.6283) (-142.4048, 85.6057) (-141.3881, 84.0523) (-140.6468, 82.2521) (-139.9554, 80.5733) (-139.4675, 78.6373) (-138.9195, 76.7225) (-138.5808, 75.5389) (-138.2149, 74.3638) (-137.8326, 73.4325) (-137.7208, 73.1603) (-137.6088, 72.9111) (-137.5, 72.6931) knots -1.056001 -1.056001 -1.056001 -1.056001 -1 -1 -1 -0.851292 -0.851292 -0.851292 -0.71262 -0.71262 -0.71262 -0.626906 -0.626906 -0.626906 -0.601856 -0.601856 -0.601856 -0.601856
  spline S35 degree 3 poles (-137.5, 72.6931) (-137.0881, 73.5183) (-136.6514, 74.7828) (-136.2668, 76.0817) (-135.7129, 77.9522) (-135.237, 79.9069) (-134.6002, 81.6203) (-133.9085, 83.4814) (-132.986, 85.1149) (-131.6355, 86.2591) (-131.4823, 86.3889) (-131.3242, 86.5122) (-131.1613, 86.6283) (-130.7742, 86.9044) (-130.3871, 87.1804) (-130, 87.4565) knots -0.398144 -0.398144 -0.398144 -0.398144 -0.30293 -0.30293 -0.30293 -0.165823 -0.165823 -0.165823 -0.016893 -0.016893 -0.016893 0 0 0 0.056001 0.056001 0.056001 0.056001
  spline S36 degree 3 poles (-130, 87.4565) (-129.6129, 87.1804) (-129.2258, 86.9044) (-128.8387, 86.6283) (-127.4048, 85.6057) (-126.3881, 84.0523) (-125.6468, 82.2521) (-124.9554, 80.5733) (-124.4675, 78.6373) (-123.9195, 76.7225) (-123.5808, 75.5389) (-123.2149, 74.3638) (-122.8326, 73.4325) (-122.7208, 73.1603) (-122.6088, 72.9111) (-122.5, 72.6931) knots -1.056001 -1.056001 -1.056001 -1.056001 -1 -1 -1 -0.851292 -0.851292 -0.851292 -0.71262 -0.71262 -0.71262 -0.626906 -0.626906 -0.626906 -0.601856 -0.601856 -0.601856 -0.601856
  spline S37 degree 3 poles (-122.5, 72.6931) (-122.0881, 73.5183) (-121.6514, 74.7828) (-121.2668, 76.0817) (-120.7129, 77.9522) (-120.237, 79.9069) (-119.6002, 81.6203) (-118.9085, 83.4814) (-117.986, 85.1149) (-116.6355, 86.2591) (-116.4823, 86.3889) (-116.3242, 86.5122) (-116.1613, 86.6283) (-115.7742, 86.9044) (-115.3871, 87.1804) (-115, 87.4565) knots -0.398144 -0.398144 -0.398144 -0.398144 -0.30293 -0.30293 -0.30293 -0.165823 -0.165823 -0.165823 -0.016893 -0.016893 -0.016893 0 0 0 0.056001 0.056001 0.056001 0.056001
  spline S38 degree 3 poles (-115, 87.4565) (-114.6129, 87.1804) (-114.2258, 86.9044) (-113.8387, 86.6283) (-112.4048, 85.6057) (-111.3881, 84.0523) (-110.6468, 82.2521) (-109.9554, 80.5733) (-109.4675, 78.6373) (-108.9195, 76.7225) (-108.5808, 75.5389) (-108.2149, 74.3638) (-107.8326, 73.4325) (-107.7208, 73.1603) (-107.6088, 72.9111) (-107.5, 72.6931) knots -1.056001 -1.056001 -1.056001 -1.056001 -1 -1 -1 -0.851292 -0.851292 -0.851292 -0.71262 -0.71262 -0.71262 -0.626906 -0.626906 -0.626906 -0.601856 -0.601856 -0.601856 -0.601856
  spline S39 degree 3 poles (-107.5, 72.6931) (-107.0881, 73.5183) (-106.6514, 74.7828) (-106.2668, 76.0817) (-105.7129, 77.9522) (-105.237, 79.9069) (-104.6002, 81.6203) (-103.9085, 83.4814) (-102.986, 85.1149) (-101.6355, 86.2591) (-101.4823, 86.3889) (-101.3242, 86.5122) (-101.1613, 86.6283) (-100.7742, 86.9044) (-100.3871, 87.1804) (-100, 87.4565) knots -0.398144 -0.398144 -0.398144 -0.398144 -0.30293 -0.30293 -0.30293 -0.165823 -0.165823 -0.165823 -0.016893 -0.016893 -0.016893 0 0 0 0.056001 0.056001 0.056001 0.056001
  spline S40 degree 3 poles (-100, 87.4565) (-99.6129, 87.1804) (-99.2258, 86.9044) (-98.8387, 86.6283) (-97.4048, 85.6057) (-96.3881, 84.0523) (-95.6468, 82.2521) (-94.9554, 80.5733) (-94.4675, 78.6373) (-93.9195, 76.7225) (-93.5808, 75.5389) (-93.2149, 74.3638) (-92.8326, 73.4325) (-92.7208, 73.1603) (-92.6088, 72.9111) (-92.5, 72.6931) knots -1.056001 -1.056001 -1.056001 -1.056001 -1 -1 -1 -0.851292 -0.851292 -0.851292 -0.71262 -0.71262 -0.71262 -0.626906 -0.626906 -0.626906 -0.601856 -0.601856 -0.601856 -0.601856
  spline S41 degree 3 poles (-92.5, 72.6931) (-92.0881, 73.5183) (-91.6514, 74.7828) (-91.2668, 76.0817) (-90.7129, 77.9522) (-90.237, 79.9069) (-89.6002, 81.6203) (-88.9085, 83.4814) (-87.986, 85.1149) (-86.6355, 86.2591) (-86.4823, 86.3889) (-86.3242, 86.5122) (-86.1613, 86.6283) (-85.7742, 86.9044) (-85.3871, 87.1804) (-85, 87.4565) knots -0.398144 -0.398144 -0.398144 -0.398144 -0.30293 -0.30293 -0.30293 -0.165823 -0.165823 -0.165823 -0.016893 -0.016893 -0.016893 0 0 0 0.056001 0.056001 0.056001 0.056001
  spline S42 degree 3 poles (-85, 87.4565) (-84.6129, 87.1804) (-84.2258, 86.9044) (-83.8387, 86.6283) (-82.4048, 85.6057) (-81.3881, 84.0523) (-80.6468, 82.2521) (-79.9554, 80.5733) (-79.4675, 78.6373) (-78.9195, 76.7225) (-78.5808, 75.5389) (-78.2149, 74.3638) (-77.8326, 73.4325) (-77.7208, 73.1603) (-77.6088, 72.9111) (-77.5, 72.6931) knots -1.056001 -1.056001 -1.056001 -1.056001 -1 -1 -1 -0.851292 -0.851292 -0.851292 -0.71262 -0.71262 -0.71262 -0.626906 -0.626906 -0.626906 -0.601856 -0.601856 -0.601856 -0.601856
  spline S43 degree 3 poles (-77.5, 72.6931) (-77.0881, 73.5183) (-76.6514, 74.7828) (-76.2668, 76.0817) (-75.7129, 77.9522) (-75.237, 79.9069) (-74.6002, 81.6203) (-73.9085, 83.4814) (-72.986, 85.1149) (-71.6355, 86.2591) (-71.4823, 86.3889) (-71.3242, 86.5122) (-71.1613, 86.6283) (-70.7742, 86.9044) (-70.3871, 87.1804) (-70, 87.4565) knots -0.398144 -0.398144 -0.398144 -0.398144 -0.30293 -0.30293 -0.30293 -0.165823 -0.165823 -0.165823 -0.016893 -0.016893 -0.016893 0 0 0 0.056001 0.056001 0.056001 0.056001
  spline S44 degree 3 poles (-70, 87.4565) (-69.6129, 87.1804) (-69.2258, 86.9044) (-68.8387, 86.6283) (-67.4048, 85.6057) (-66.3881, 84.0523) (-65.6468, 82.2521) (-64.9554, 80.5733) (-64.4675, 78.6373) (-63.9195, 76.7225) (-63.5808, 75.5389) (-63.2149, 74.3638) (-62.8326, 73.4325) (-62.7208, 73.1603) (-62.6088, 72.9111) (-62.5, 72.6931) knots -1.056001 -1.056001 -1.056001 -1.056001 -1 -1 -1 -0.851292 -0.851292 -0.851292 -0.71262 -0.71262 -0.71262 -0.626906 -0.626906 -0.626906 -0.601856 -0.601856 -0.601856 -0.601856
  spline S45 degree 3 poles (-62.5, 72.6931) (-62.0881, 73.5183) (-61.6514, 74.7828) (-61.2668, 76.0817) (-60.7129, 77.9522) (-60.237, 79.9069) (-59.6002, 81.6203) (-58.9085, 83.4814) (-57.986, 85.1149) (-56.6355, 86.2591) (-56.4823, 86.3889) (-56.3242, 86.5122) (-56.1613, 86.6283) (-55.7742, 86.9044) (-55.3871, 87.1804) (-55, 87.4565) knots -0.398144 -0.398144 -0.398144 -0.398144 -0.30293 -0.30293 -0.30293 -0.165823 -0.165823 -0.165823 -0.016893 -0.016893 -0.016893 0 0 0 0.056001 0.056001 0.056001 0.056001
  spline S46 degree 3 poles (-55, 87.4565) (-54.6129, 87.1804) (-54.2258, 86.9044) (-53.8387, 86.6283) (-52.4048, 85.6057) (-51.3881, 84.0523) (-50.6468, 82.2521) (-49.9554, 80.5733) (-49.4675, 78.6373) (-48.9195, 76.7225) (-48.5808, 75.5389) (-48.2149, 74.3638) (-47.8326, 73.4325) (-47.7208, 73.1603) (-47.6088, 72.9111) (-47.5, 72.6931) knots -1.056001 -1.056001 -1.056001 -1.056001 -1 -1 -1 -0.851292 -0.851292 -0.851292 -0.71262 -0.71262 -0.71262 -0.626906 -0.626906 -0.626906 -0.601856 -0.601856 -0.601856 -0.601856
  spline S47 degree 3 poles (-47.5, 72.6931) (-47.0881, 73.5183) (-46.6514, 74.7828) (-46.2668, 76.0817) (-45.7129, 77.9522) (-45.237, 79.9069) (-44.6002, 81.6203) (-43.9085, 83.4814) (-42.986, 85.1149) (-41.6355, 86.2591) (-41.4823, 86.3889) (-41.3242, 86.5122) (-41.1613, 86.6283) (-40.7742, 86.9044) (-40.3871, 87.1804) (-40, 87.4565) knots -0.398144 -0.398144 -0.398144 -0.398144 -0.30293 -0.30293 -0.30293 -0.165823 -0.165823 -0.165823 -0.016893 -0.016893 -0.016893 0 0 0 0.056001 0.056001 0.056001 0.056001
  arc A18 (-9.9941, 94.9941) -> (-10.0059, 95) centre (-12.5, 89.9985) ccw
  arc A19 (-14.994, 95) -> (-15.006, 94.994) centre (-12.5, 89.9985) ccw
  line L29 (-2.3166, 87.5) -> (-7.5007, 87.5)
  line L30 (-17.4992, 87.5) -> (-20.5, 87.5)
  arc A20 (-20.5, 97) -> (-20.5, 87.5) centre (-20.5, 92.25) ccw
  spline S48 degree 3 poles (-8.3546, 86.25) (-7.1718, 85.2406) (-6.3018, 83.8427) (-5.6468, 82.2521) (-4.9928, 80.664) (-4.5209, 78.846) (-4.0079, 77.0332) knots -0.982686 -0.982686 -0.982686 -0.982686 -0.851293 -0.851293 -0.851293 -0.720109 -0.720109 -0.720109 -0.720109
  spline S49 degree 3 poles (-17.5, 72.6931) (-17.0881, 73.5183) (-16.6514, 74.7828) (-16.2668, 76.0817) (-15.7129, 77.9522) (-15.237, 79.9069) (-14.6002, 81.6203) (-14.2177, 82.6495) (-13.7647, 83.609) (-13.2077, 84.4547) knots -0.398144 -0.398144 -0.398144 -0.398144 -0.30293 -0.30293 -0.30293 -0.165823 -0.165823 -0.165823 -0.083469 -0.083469 -0.083469 -0.083469
  arc A21 (-17.4992, 87.5) -> (-13.2077, 84.4547) centre (-12.5, 89.9985) ccw
  arc A22 (-8.3546, 86.25) -> (-7.5007, 87.5) centre (-12.5, 89.9985) ccw
  line L31 (-252.4773, 87.4565) -> (-257.6718, 87.4565)
  line L32 (-239.4991, 87.4565) -> (-242.5226, 87.4565)
  arc A23 (-239.4991, 87.4565) -> (-239.5, 97) centre (-239.547, 92.2282) ccw
  spline S50 degree 3 poles (-246.7932, 84.4545) (-246.3501, 83.7838) (-245.9719, 83.0417) (-245.6468, 82.2521) (-244.9554, 80.5733) (-244.4675, 78.6373) (-243.9195, 76.7225) (-243.5808, 75.5389) (-243.2149, 74.3638) (-242.8326, 73.4325) (-242.7208, 73.1603) (-242.6088, 72.9111) (-242.5, 72.6931) knots -0.916519 -0.916519 -0.916519 -0.916519 -0.851292 -0.851292 -0.851292 -0.71262 -0.71262 -0.71262 -0.626906 -0.626906 -0.626906 -0.601856 -0.601856 -0.601856 -0.601856
  arc A24 (-246.7932, 84.4545) -> (-242.5226, 87.4565) centre (-247.5, 89.9985) ccw
  spline S51 degree 3 poles (-255.8863, 77.4088) (-255.8862, 77.4091) (-255.8861, 77.4095) (-255.886, 77.4098) (-255.8058, 77.6957) (-255.7255, 77.9842) (-255.644, 78.2748) (-255.5645, 78.558) (-255.4839, 78.8436) (-255.4008, 79.1313) (-255.3205, 79.4094) (-255.2379, 79.6899) (-255.1515, 79.9724) (-255.0686, 80.2437) (-254.9821, 80.5174) (-254.8905, 80.7929) (-254.803, 81.0561) (-254.7107, 81.3216) (-254.6119, 81.5886) (-254.5179, 81.8428) (-254.4179, 82.099) (-254.31, 82.3561) (-254.2075, 82.6004) (-254.0979, 82.8461) (-253.9792, 83.0921) (-253.8665, 83.3255) (-253.7455, 83.5596) (-253.6145, 83.793) (-253.49, 84.0146) (-253.3563, 84.236) (-253.2115, 84.4554) (-253.0738, 84.6642) (-252.926, 84.8714) (-252.7666, 85.0751) (-252.6143, 85.2699) (-252.4515, 85.4614) (-252.2772, 85.6476) (-252.1094, 85.8267) (-251.9312, 86.0006) (-251.7418, 86.1673) (-251.7101, 86.1952) (-251.6781, 86.223) (-251.6457, 86.2504) knots -0.921631 -0.921631 -0.921631 -0.921631 -0.921529 -0.921529 -0.921529 -0.831696 -0.831696 -0.831696 -0.744179 -0.744179 -0.744179 -0.659582 -0.659582 -0.659582 -0.578332 -0.578332 -0.578332 -0.500694 -0.500694 -0.500694 -0.426786 -0.426786 -0.426786 -0.356594 -0.356594 -0.356594 -0.289994 -0.289994 -0.289994 -0.226758 -0.226758 -0.226758 -0.166571 -0.166571 -0.166571 -0.109035 -0.109035 -0.109035 -0.053684 -0.053684 -0.053684 -0.044405 -0.044405 -0.044405 -0.044405
  arc A25 (-252.4773, 87.4565) -> (-251.6457, 86.2504) centre (-247.5, 89.9985) ccw
  arc A26 (-249.9941, 95) -> (-250.0059, 94.9941) centre (-247.5, 89.9985) ccw
  arc A27 (-244.9942, 94.9942) -> (-245.0058, 95) centre (-247.5, 89.9985) ccw
  constraint concentric A14 A16
  constraint concentric A13 A17
  constraint concentric A2 A18
  constraint coincident S16.end A18
  constraint coincident L3 A18.start
  constraint coincident L2 A18.end
  constraint coincident L2 A19.start
  constraint concentric A18 A19
  constraint coincident L1 A19.end
  constraint parallel L29 L30
  constraint tangent L28 A20
  constraint coincident L28 A20.start
  constraint coincident S48.start A21
  constraint concentric A21 A22
  constraint horizontal L31
  constraint parallel L31 L32
  constraint coincident L28 A23.end
  constraint coincident L19 A26.end
  constraint coincident L20 A27.end
  constraint coincident L20 A26.start
  constraint coincident L21 A27.start